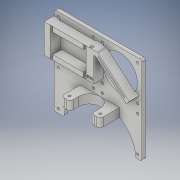
# Autodesk Inventor part: 30_LS_Sample_stage_v2
Saved by Autodesk Inventor 2019 (Build 230136000, 136)
## iProperties
Created: 2020-06-11
Part Number: 30_LS_Sample_stage_v2
Material: Generic
Document SubType Name: Modeling
Designer: UC2
Density: 1 g/cm^3
Appearance: Default
Author: UC2
Autodesk Inventor part; units mm, degrees
ref_plane "YZ Plane" through (0, 0, 0) normal (1, 0, 0) x (0, 1, 0)
ref_plane "XZ Plane" through (0, 0, 0) normal (0, 1, 0) x (-1, 0, 0)
ref_plane "XY Plane" through (0, 0, 0) normal (0, 0, 1) x (1, 0, 0)
sketch "Skizze1" plane through (0, 0, 0) normal (0, 0, 1) x (1, 0, 0)
  line L0 (9.1, 17.5) -> (9.1, 25) construction
  line L1 (9.1, 17.5) -> (15.5, 17.5) construction
  arc A0 (17.5, 15.5) -> (15.5, 17.5) centre (15.5, 15.5) ccw construction
  line L2 (17.5, 15.5) -> (17.5, 9.1) construction
  line L3 (25, 9.1) -> (17.5, 9.1) construction
  line L4 (25, 9.1) -> (25, 25) construction
  line L5 (25, 25) -> (9.1, 25) construction
  circle A1 centre (20, 20) radius 2.2989 construction
  line L6 (-9.1, 25) -> (-9.1, 17.5) construction
  line L7 (-9.1, 25) -> (-25, 25) construction
  line L8 (-25, 25) -> (-25, 9.1) construction
  line L9 (-17.5, 9.1) -> (-25, 9.1) construction
  line L10 (-17.5, 9.1) -> (-17.5, 15.5) construction
  arc A2 (-15.5, 17.5) -> (-17.5, 15.5) centre (-15.5, 15.5) ccw construction
  line L11 (-15.5, 17.5) -> (-9.1, 17.5) construction
  circle A3 centre (-20, 20) radius 2.2989 construction
  circle A4 centre (-20, -20) radius 2.2989 construction
  line L12 (-25, -9.1) -> (-17.5, -9.1) construction
  line L13 (-25, -9.1) -> (-25, -25) construction
  line L14 (-25, -25) -> (-9.1, -25) construction
  line L15 (-9.1, -17.5) -> (-9.1, -25) construction
  line L16 (-9.1, -17.5) -> (-15.5, -17.5) construction
  arc A5 (-17.5, -15.5) -> (-15.5, -17.5) centre (-15.5, -15.5) ccw construction
  line L17 (-17.5, -15.5) -> (-17.5, -9.1) construction
  line L18 (9.1, -25) -> (9.1, -17.5) construction
  line L19 (9.1, -25) -> (25, -25) construction
  line L20 (25, -25) -> (25, -9.1) construction
  line L21 (17.5, -9.1) -> (25, -9.1) construction
  line L22 (17.5, -9.1) -> (17.5, -15.5) construction
  arc A6 (15.5, -17.5) -> (17.5, -15.5) centre (15.5, -15.5) ccw construction
  line L23 (15.5, -17.5) -> (9.1, -17.5) construction
  circle A7 centre (20, -20) radius 2.2989 construction
  circle A8 centre (30, -20) radius 2.2989 construction
  line L24 (25, -9.1) -> (32.5, -9.1) construction
  line L25 (25, -9.1) -> (25, -25) construction
  line L26 (25, -25) -> (40.9, -25) construction
  line L27 (40.9, -17.5) -> (40.9, -25) construction
  line L28 (40.9, -17.5) -> (34.5, -17.5) construction
  arc A9 (32.5, -15.5) -> (34.5, -17.5) centre (34.5, -15.5) ccw construction
  line L29 (32.5, -15.5) -> (32.5, -9.1) construction
  line L30 (40.9, 25) -> (40.9, 17.5) construction
  line L31 (40.9, 25) -> (25, 25) construction
  line L32 (25, 25) -> (25, 9.1) construction
  line L33 (32.5, 9.1) -> (25, 9.1) construction
  line L34 (32.5, 9.1) -> (32.5, 15.5) construction
  arc A10 (34.5, 17.5) -> (32.5, 15.5) centre (34.5, 15.5) ccw construction
  line L35 (34.5, 17.5) -> (40.9, 17.5) construction
  circle A11 centre (30, 20) radius 2.2989 construction
  line L36 (59.1, 17.5) -> (59.1, 25) construction
  line L37 (59.1, 17.5) -> (65.5, 17.5) construction
  arc A12 (67.5, 15.5) -> (65.5, 17.5) centre (65.5, 15.5) ccw construction
  line L38 (67.5, 15.5) -> (67.5, 9.1) construction
  line L39 (75, 9.1) -> (67.5, 9.1) construction
  line L40 (75, 9.1) -> (75, 25) construction
  line L41 (75, 25) -> (59.1, 25) construction
  circle A13 centre (70, 20) radius 2.2989 construction
  line L42 (59.1, -25) -> (59.1, -17.5) construction
  line L43 (59.1, -25) -> (75, -25) construction
  line L44 (75, -25) -> (75, -9.1) construction
  line L45 (67.5, -9.1) -> (75, -9.1) construction
  line L46 (67.5, -9.1) -> (67.5, -15.5) construction
  arc A14 (65.5, -17.5) -> (67.5, -15.5) centre (65.5, -15.5) ccw construction
  line L47 (65.5, -17.5) -> (59.1, -17.5) construction
  circle A15 centre (70, -20) radius 2.2989 construction
  line L48 (213.1196, -154.9196) -> (-182.4616, 240.6616) construction
  line L49 (-24.9, 24.9) -> (74.7, 24.9)
  line L50 (74.7, 24.9) -> (74.7, -74.7)
  line L51 (74.7, -74.7) -> (-24.9, -74.7)
  line L52 (-24.9, -74.7) -> (-24.9, 24.9)
  circle A16 centre (50, 0) radius 19.7246
  point P0 (0, 0)
  dimension "d0" = 99.6
  dimension "d1" = 99.6
  dimension "d2" = 0.1
  dimension "d3" = 0.1
  constraints: 10 end point, 2 parallel, 1 coincident, 1 horizontal, 1 perpendicular, 6 other
  measures "d0" distance of L51.end L49.start
  measures "d1" distance of L50.end L51.end
  measures "d2" distance between parallel lines of L8 L52
  measures "d3" distance between parallel lines of L7 L49
extrude "Extrusion1" add sketch "Skizze1" along normal blind 4
sketch "Skizze2" plane through (0, 0, 0) normal (0, 0, -1) x (-1, 0, 0)
  circle A0 centre (20, -20) radius 2.1796 construction
  circle A1 centre (20, 20) radius 2.1796 construction
  circle A2 centre (-20, 20) radius 2.1796 construction
  circle A3 centre (-20, -20) radius 2.1796 construction
  circle A4 centre (-30, -20) radius 2.1796 construction
  circle A5 centre (-70, -20) radius 2.1796 construction
  circle A6 centre (-70, 20) radius 2.1796 construction
  circle A7 centre (-30, 20) radius 2.1796 construction
  circle A8 centre (-70, -70) radius 2.65 construction
  circle A9 centre (-30, -70) radius 2.65 construction
  circle A10 centre (-20, -70) radius 2.65 construction
  circle A11 centre (20, -70) radius 2.65 construction
  circle A12 centre (20, -30) radius 2.65 construction
  circle A13 centre (-20, -30) radius 2.65 construction
  circle A14 centre (-30, -30) radius 2.65 construction
  circle A15 centre (-70, -30) radius 2.65 construction
  point P0 (0, 0)
hole "Bohrung1" at (-20, -20, 0) at (-20, 20, 0) at (20, -20, 0) at (30, -20, 0) at (70, -20, 0) at (70, 20, 0) at (30, 20, 0) at (20, 20, 0) at (70, -30, 0) at (30, -30, 0) at (20, -30, 0) at (-20, -30, 0) at (-20, -70, 0) at (20, -70, 0) at (30, -70, 0) at (70, -70, 0) direction (0, 0, 1) diameter 2.8 end through all
ref_plane "Arbeitsebene1" through (0, 0, 5.25) normal (0, 0, 1) x (1, 0, 0)
sketch "Skizze4" plane through (0, 0, 5.25) normal (0, 0, 1) x (1, 0, 0)
  line L0 (-24.9, 24.9) -> (-24.9, -74.7) construction
  line L1 (-24.9, -74.7) -> (74.7, -74.7) construction
  line L2 (74.7, -74.7) -> (74.7, 24.9) construction
  line L3 (74.7, 24.9) -> (-24.9, 24.9) construction
  circle A0 centre (30, 20) radius 1.4 construction
  circle A1 centre (70, -20) radius 1.4 construction
  circle A2 centre (20, -20) radius 1.4 construction
  circle A3 centre (-20, -20) radius 1.4 construction
  circle A4 centre (-20, 20) radius 1.4 construction
  circle A5 centre (30, -20) radius 1.4 construction
  circle A6 centre (70, 20) radius 1.4 construction
  circle A7 centre (20, 20) radius 1.4 construction
  circle A8 centre (51.5846, 1.8884) radius 19.7246 construction
  circle A9 centre (70, -20) radius 1.4 construction
  line L4 (-24.9, 18.6) -> (-17.9, 18.6)
  line L5 (-17.9, 18.6) -> (-17.9, -14.4)
  line L6 (-17.9, -14.4) -> (-24.9, -14.4)
  line L7 (-24.9, -14.4) -> (-24.9, 18.6)
  line L8 (31.6685, 18.6) -> (22.6685, 18.6)
  line L9 (22.6685, 18.6) -> (22.6685, -14.4)
  line L10 (22.6685, -14.4) -> (31.6685, -14.4)
  line L11 (31.6685, -14.4) -> (31.6685, 18.6)
  line L12 (-17.9, 18.6) -> (22.6685, 18.6)
  line L13 (22.6685, 18.6) -> (22.6685, 18.1)
  line L14 (22.6685, 18.1) -> (-17.9, 18.1)
  line L15 (-17.9, 18.1) -> (-17.9, 18.6)
  line L16 (-17.9, -14.4) -> (22.6685, -14.4)
  line L17 (22.6685, -14.4) -> (22.6685, -13.9)
  line L18 (22.6685, -13.9) -> (-17.9, -13.9)
  line L19 (-17.9, -13.9) -> (-17.9, -14.4)
  line L20 (-14.9, -13.9) -> (19.6685, -13.9)
  line L21 (19.6685, -13.9) -> (19.6685, -8.9)
  line L22 (19.6685, -8.9) -> (-14.9, -8.9)
  line L23 (-14.9, -8.9) -> (-14.9, -13.9)
  line L24 (-14.9, 18.1) -> (19.6685, 18.1)
  line L25 (19.6685, 18.1) -> (19.6685, 13.1)
  line L26 (19.6685, 13.1) -> (-14.9, 13.1)
  line L27 (-14.9, 13.1) -> (-14.9, 18.1)
  line L28 (22.6685, 18.6) -> (31.6685, 18.6)
  line L29 (31.6685, 18.6) -> (31.6685, -14.4)
  line L30 (31.6685, -14.4) -> (22.6685, -14.4)
  line L31 (22.6685, -14.4) -> (22.6685, 18.6)
  line L32 (30, 20) -> (73.3204, -16.3501) construction
  line L33 (31.6685, 18.6) -> (34.9854, 18.6)
  line L34 (36.271, 18.1321) -> (71.6704, -11.5715)
  line L35 (71.6704, -11.5715) -> (68.3279, -15.555)
  line L36 (68.3279, -15.555) -> (34.14, 13.1321)
  line L37 (32.8544, 13.6) -> (31.6685, 13.6)
  line L38 (66.3088, -11.25) -> (36.089, 14.1075)
  line L39 (36.089, 14.1075) -> (36.8603, 15.0268)
  line L40 (36.8603, 15.0268) -> (67.0802, -10.3307)
  line L41 (67.0802, -10.3307) -> (66.3088, -11.25)
  line L42 (66.3088, -11.25) -> (36.8603, 15.0268) construction
  line L43 (36.089, 14.1075) -> (67.0802, -10.3307) construction
  arc A10 (34.14, 13.1321) -> (32.8544, 13.6) centre (32.8544, 11.6) ccw
  arc A11 (36.271, 18.1321) -> (34.9854, 18.6) centre (34.9854, 16.6) ccw
  line L44 (31.6685, 13.6) -> (31.6685, 18.6)
  line L45 (30, 20) -> (70, 20) construction
  point P0 (0, 0)
  point P1 (51.5846, 1.8884)
  dimension "d15" = 5
  dimension "d16" = 5
  dimension "d17" = 3
  dimension "d18" = 3
  dimension "d19" = 0.5
  dimension "d20" = 0.5
  dimension "d21" = 7
  dimension "d22" = 9
  dimension "d70" = 33
  dimension "d71" = 5
  dimension "d73" = 1.2
  dimension "d74" = 2
  dimension "d75" = 5.2
  dimension "d95" = 40
  constraints: 84 end point, 20 parallel, 12 point on line, 9 horizontal, 9 perpendicular, 5 tangent, 4 point on circle, 3 centre point, 3 midpoint, 1 coincident, 1 collinear, 1 equal radius, 1 other
  measures "d15" distance of L26.end L24.start
  measures "d16" distance of L22.end L20.start
  measures "d17" distance between parallel lines of L5 L23
  measures "d18" distance between parallel lines of L9 L21
  measures "d19" distance between parallel lines of L16 L18
  measures "d20" distance between parallel lines of L14 L12
  measures "d21" distance of L4.start L4.end
  measures "d22" distance of L8.start L8.end
  measures "d70" distance of L4.end L5.end
  measures "d71" distance between parallel lines of L33 L37
  measures "d73" distance of L38.end L39.end
  measures "d74" radius of A10
  measures "d75" distance of L34.end L35.end
  measures "d95" angle of L32 L45
extrude "Extrusion2" add sketch "Skizze4" along normal blind 20 contours L4 L5 L6 L7 | L12 L9 L14 L5 | L8 L11 L10 L9 | L5 L18 L9 L16 | L14 L25 L26 L27 | L33 A11 L34 L35 L36 A10 L37 L11 | L23 L22 L21 L18
sketch "Skizze5" plane through (0, 0, 4) normal (0, 0, 1) x (1, 0, 0)
  line L0 (-24.9, -14.4) -> (31.6685, -14.4) construction
  line L1 (34.9854, 18.6) -> (-24.9, 18.6) construction
  line L2 (-24.9, 18.6) -> (-24.9, -14.4) construction
  line L3 (-17.9, -13.9) -> (-17.9, 18.1) construction
  line L4 (-17.9, 18.1) -> (-14.9, 18.1) construction
  line L5 (-14.9, 18.1) -> (-14.9, 13.1) construction
  line L6 (-14.9, 13.1) -> (19.6685, 13.1) construction
  line L7 (19.6685, 13.1) -> (19.6685, 18.1) construction
  line L8 (19.6685, 18.1) -> (22.6685, 18.1) construction
  line L9 (22.6685, -13.9) -> (19.6685, -13.9) construction
  line L10 (19.6685, -13.9) -> (19.6685, -8.9) construction
  line L11 (19.6685, -8.9) -> (-14.9, -8.9) construction
  line L12 (-14.9, -8.9) -> (-14.9, -13.9) construction
  line L13 (-14.9, -13.9) -> (-17.9, -13.9) construction
  line L14 (-24.9, 18.6) -> (-17.9, 18.6)
  line L15 (-17.9, 18.6) -> (-17.9, -14.4)
  line L16 (-17.9, -14.4) -> (-24.9, -14.4)
  line L17 (-24.9, -14.4) -> (-24.9, 18.6)
  line L18 (31.6685, -14.4) -> (31.6685, 13.6) projected
  line L19 (22.6685, 18.1) -> (22.6685, -13.9) projected
  line L20 (31.6685, 13.6) -> (32.8544, 13.6) projected
  arc A0 (34.14, 13.1321) -> (32.8544, 13.6) centre (32.8544, 11.6) ccw projected
  line L21 (34.14, 13.1321) -> (68.3279, -15.555) projected
  line L22 (68.3279, -15.555) -> (71.6704, -11.5715) projected
  line L23 (71.6704, -11.5715) -> (36.271, 18.1321) projected
  arc A1 (36.271, 18.1321) -> (34.9854, 18.6) centre (34.9854, 16.6) ccw projected
  point P0 (0, 0)
  constraints: 8 end point, 2 parallel, 1 horizontal, 1 perpendicular, 1 point on line
extrude "Extrusion3" add sketch "Skizze5" along normal up to next
sketch "Skizze9" plane through (0, 0, 4) normal (0, 0, 1) x (1, 0, 0)
  line L0 (74.7, -74.7) -> (74.7, 24.9) construction
  line L1 (74.7, 24.9) -> (-24.9, 24.9) construction
  line L2 (-24.9, -14.4) -> (-24.9, -74.7) construction
  line L3 (-24.9, 18.6) -> (-20, 18.6) construction
  line L4 (-17.9, 18.6) -> (-17.9, -14.4) construction
  line L5 (-17.9, -14.4) -> (-24.9, -14.4) construction
  line L6 (-24.9, 24.9) -> (-24.9, 18.6) construction
  circle A0 centre (30, 20) radius 1.4 construction
  circle A1 centre (70, -20) radius 1.4 construction
  circle A2 centre (20, -20) radius 1.4 construction
  circle A3 centre (-20, -20) radius 1.4 construction
  circle A4 centre (-20, 20) radius 1.4 construction
  circle A5 centre (30, -20) radius 1.4 construction
  circle A6 centre (70, 20) radius 1.4 construction
  circle A7 centre (20, 20) radius 1.4 construction
  circle A8 centre (50, 0) radius 19.7246 construction
  line L7 (34.9854, 18.6) -> (-24.9, 18.6) construction
  line L8 (-24.9, 18.6) -> (-24.9, -14.4) construction
  line L9 (-24.9, -14.4) -> (31.6685, -14.4) construction
  line L10 (-17.9, 18.1) -> (-14.9, 18.1) construction
  line L11 (-14.9, 18.1) -> (-14.9, 13.1) construction
  line L12 (-14.9, 13.1) -> (19.6685, 13.1) construction
  line L13 (19.6685, 13.1) -> (19.6685, 18.1) construction
  line L14 (19.6685, 18.1) -> (22.6685, 18.1) construction
  line L15 (22.6685, -13.9) -> (19.6685, -13.9) construction
  line L16 (19.6685, -13.9) -> (19.6685, -8.9) construction
  line L17 (19.6685, -8.9) -> (-14.9, -8.9) construction
  line L18 (-14.9, -8.9) -> (-14.9, -13.9) construction
  line L19 (-14.9, -13.9) -> (-17.9, -13.9) construction
  line L20 (-17.9, -13.9) -> (-17.9, 18.1) construction
  line L21 (5.1685, -34.4) -> (49.1685, -34.4)
  line L22 (49.1685, -34.4) -> (49.1685, -44.4)
  line L23 (49.1685, -44.4) -> (5.1685, -44.4)
  line L24 (5.1685, -44.4) -> (5.1685, -34.4)
  line L25 (31.6685, -14.4) -> (31.6685, 13.6) projected
  line L26 (22.6685, 18.1) -> (22.6685, -13.9) projected
  line L27 (-20, 18.6) -> (-17.9, 18.6) projected
  line L28 (31.6685, 13.6) -> (32.8544, 13.6) projected
  arc A9 (34.14, 13.1321) -> (32.8544, 13.6) centre (32.8544, 11.6) ccw projected
  line L29 (34.14, 13.1321) -> (68.3279, -15.555) projected
  line L30 (68.3279, -15.555) -> (71.6704, -11.5715) projected
  line L31 (71.6704, -11.5715) -> (36.271, 18.1321) projected
  arc A10 (36.271, 18.1321) -> (34.9854, 18.6) centre (34.9854, 16.6) ccw projected
  line L32 (27.1685, 18.6) -> (27.1685, -74.7) construction
  line L33 (74.7, -74.7) -> (-24.9, -74.7) construction
  line L34 (-24.9, -74.7) -> (74.7, -74.7) projected
  point P0 (0, 0)
  dimension "d44" = 10
  dimension "d45" = 20
  dimension "d53" = 44
  dimension "d80" = 4.5
  constraints: 10 end point, 2 parallel, 2 point on line, 1 horizontal, 1 perpendicular, 1 vertical, 1 vertical alignment, 1 other
  measures "d44" distance of L23.end L21.start
  measures "d45" distance between parallel lines of L9 L21
  measures "d53" distance of L22.end L23.end
  measures "d80" distance between parallel lines of L26 L32
extrude "Extrusion6" add sketch "Skizze9" along normal blind 22
sketch "Skizze10" plane through (5.1685, -44.4, 4) normal (0, -1, 0) x (1, 0, 0)
  circle A0 centre (4.5, 17) radius 2.1 construction
  circle A1 centre (39.5, 17) radius 2.1 construction
  circle A2 centre (22, 6.652) radius 4.55 construction
  circle A3 centre (4.5, 17) radius 1.4
  circle A4 centre (39.5, 17) radius 1.4
  line L0 (29.8169, 1.25) -> (-23.0685, 1.25) projected
  line L1 (44, 0) -> (0, 0) construction
  line L2 (44, 0) -> (44, 22) construction
  line L3 (0, 22) -> (44, 22) construction
  line L4 (0, 0) -> (0, 22) construction
  line L5 (0, 22) -> (44, 22) construction
  line L6 (22, 22) -> (22, -2.1382) construction
  line L7 (22, 12) -> (22, 21.4772) construction
  line L8 (34, 12) -> (34, 21.4772)
  line L9 (10, 21.4772) -> (10, 12)
  arc A5 (10, 12) -> (34, 12) centre (22, 12) ccw
  arc A6 (34, 21.4772) -> (10, 21.4772) centre (22, 21.4772) ccw
  point P0 (-5.1685, -4)
  point P1 (56.4063, 1.25)
  point P2 (3.1, 1.25)
  point P3 (22, 16.7386)
  point P4 (50.2492, 1.25)
  point P5 (4.1, 1.25)
  dimension "d48" = 2.8
  dimension "d49" = 2.8
  dimension "d54" = 35
  dimension "d65" = 24
  dimension "d78" = 5
  constraints: 10 end point, 7 centre point, 5 tangent, 4 point on circle, 3 point on line, 2 coincident, 2 midpoint, 1 parallel, 1 perpendicular, 1 symmetric about line
  measures "d48" diameter of A3
  measures "d49" diameter of A4
  measures "d54" distance of A0.centre A1.centre
  measures "d65" distance between parallel lines of L9 L8
  measures "d78" distance from line of L3 A0.centre
extrude "Extrusion7" cut sketch "Skizze10" against normal up to surface (10 mm away)
fillet "Rundung3" radius 3.5 4 edges at (49.1685, -39.4, 26) (5.1685, -39.4, 26) (15.1798, -39.4, 26) (39.1571, -39.4, 26)
sketch "Skizze15" plane through (-17.9, -14.4, 5.25) normal (0, -1, 0) x (1, 0, 0)
  line L0 (0, -1.25) -> (0, 0) construction
  line L1 (0, 0) -> (49.5685, 0) construction
  line L2 (49.5685, 0) -> (49.5685, 20) construction
  line L3 (-7, 20) -> (49.5685, 20) construction
  line L4 (-7, -1.25) -> (-7, 20) projected
  line L5 (0, -1.25) -> (-7, -1.25) projected
  line L6 (44.7786, 9.164) -> (46.148, 8.708) construction
  line L7 (46.148, 8.708) -> (46.4379, 7.2941) construction
  line L8 (46.4379, 7.2941) -> (45.3583, 6.336) construction
  line L9 (45.3583, 6.336) -> (43.9889, 6.792) construction
  line L10 (43.9889, 6.792) -> (43.699, 8.2059) construction
  line L11 (43.699, 8.2059) -> (44.7786, 9.164) construction
  circle A0 centre (45.0685, 7.75) radius 2.45 construction
  point P0 (17.9, -5.25)
hole "Bohrung3" at (27.1685, -14.4, 13) direction (0, 1, 0) diameter 3.5 end through all
sketch "Skizze16" plane through (0, 0, 25.25) normal (0, 0, 1) x (1, 0, 0)
  line L0 (25.4185, 18.6) -> (25.4185, -14.4) construction
  line L1 (28.9185, 18.6) -> (28.9185, -14.4) construction
  line L2 (-17.9, 18.1) -> (-14.9, 18.1) construction
  line L3 (-14.9, 18.1) -> (-14.9, 13.1) construction
  line L4 (-14.9, 13.1) -> (19.6685, 13.1) construction
  line L5 (19.6685, 13.1) -> (19.6685, 18.1) construction
  line L6 (19.6685, 18.1) -> (22.6685, 18.1) construction
  line L7 (22.6685, 18.1) -> (22.6685, -13.9) construction
  line L8 (22.6685, -13.9) -> (19.6685, -13.9) construction
  line L9 (19.6685, -13.9) -> (19.6685, -8.9) construction
  line L10 (19.6685, -8.9) -> (-14.9, -8.9) construction
  line L11 (-14.9, -8.9) -> (-14.9, -13.9) construction
  line L12 (-14.9, -13.9) -> (-17.9, -13.9) construction
  line L13 (-17.9, -13.9) -> (-17.9, 18.1) construction
  line L14 (36.089, 14.1075) -> (36.8603, 15.0268) construction
  line L15 (36.8603, 15.0268) -> (67.0802, -10.3307) construction
  line L16 (67.0802, -10.3307) -> (66.3088, -11.25) construction
  line L17 (66.3088, -11.25) -> (36.089, 14.1075) construction
  line L18 (34.9854, 18.6) -> (-24.9, 18.6) construction
  line L19 (-24.9, -14.4) -> (31.6685, -14.4) construction
  line L20 (31.6685, -14.4) -> (31.6685, 13.6) construction
  line L21 (31.6685, 13.6) -> (32.8544, 13.6) construction
  arc A0 (34.14, 13.1321) -> (32.8544, 13.6) centre (32.8544, 11.6) ccw construction
  line L22 (34.14, 13.1321) -> (68.3279, -15.555) construction
  line L23 (68.3279, -15.555) -> (71.6704, -11.5715) construction
  line L24 (71.6704, -11.5715) -> (36.271, 18.1321) construction
  arc A1 (36.271, 18.1321) -> (34.9854, 18.6) centre (34.9854, 16.6) ccw construction
  line L25 (28.9185, -14.4) -> (25.4185, -14.4) projected
  line L26 (27.1685, -14.4) -> (27.1685, 18.6) construction
  line L27 (34.9854, 18.6) -> (-24.9, 18.6) projected
  line L28 (23.9185, -11.8716) -> (30.4185, -11.8716)
  line L29 (30.4185, -11.8716) -> (30.4185, -9.3716)
  line L30 (30.4185, -9.3716) -> (23.9185, -9.3716)
  line L31 (23.9185, -9.3716) -> (23.9185, -11.8716)
  line L32 (-24.9, 18.6) -> (-24.9, -14.4) projected
  point P0 (0, 0)
  dimension "d88" = 2.5
  dimension "d89" = 6.5
  constraints: 10 end point, 2 parallel, 2 perpendicular, 1 horizontal, 1 midpoint, 1 point on line, 1 other
  measures "d88" distance of L28.end L29.end
  measures "d89" distance of L28.start L28.end
extrude "Extrusion12" cut sketch "Skizze16" against normal up to surface (21.25 mm away)
sketch "Skizze17" plane through (0, 0, 25.25) normal (0, 0, 1) x (1, 0, 0)
  line L0 (30.4185, -11.8716) -> (23.9185, -11.8716) construction
  line L1 (23.9185, -11.8716) -> (23.9185, -9.3716) construction
  line L2 (23.9185, -9.3716) -> (30.4185, -9.3716) construction
  line L3 (30.4185, -9.3716) -> (30.4185, -11.8716) construction
  line L4 (-17.9, 18.1) -> (-14.9, 18.1) construction
  line L5 (-14.9, 18.1) -> (-14.9, 13.1) construction
  line L6 (-14.9, 13.1) -> (19.6685, 13.1) construction
  line L7 (19.6685, 13.1) -> (19.6685, 18.1) construction
  line L8 (19.6685, 18.1) -> (22.6685, 18.1) construction
  line L9 (22.6685, 18.1) -> (22.6685, -13.9) construction
  line L10 (22.6685, -13.9) -> (19.6685, -13.9) construction
  line L11 (19.6685, -13.9) -> (19.6685, -8.9) construction
  line L12 (19.6685, -8.9) -> (-14.9, -8.9) construction
  line L13 (-14.9, -8.9) -> (-14.9, -13.9) construction
  line L14 (-14.9, -13.9) -> (-17.9, -13.9) construction
  line L15 (-17.9, -13.9) -> (-17.9, 18.1) construction
  line L16 (36.089, 14.1075) -> (36.8603, 15.0268) construction
  line L17 (36.8603, 15.0268) -> (67.0802, -10.3307) construction
  line L18 (67.0802, -10.3307) -> (66.3088, -11.25) construction
  line L19 (66.3088, -11.25) -> (36.089, 14.1075) construction
  line L20 (34.9854, 18.6) -> (-24.9, 18.6) construction
  line L21 (-24.9, -14.4) -> (31.6685, -14.4) construction
  line L22 (31.6685, -14.4) -> (31.6685, 13.6) construction
  line L23 (31.6685, 13.6) -> (32.8544, 13.6) construction
  arc A0 (34.14, 13.1321) -> (32.8544, 13.6) centre (32.8544, 11.6) ccw construction
  line L24 (34.14, 13.1321) -> (68.3279, -15.555) construction
  line L25 (68.3279, -15.555) -> (71.6704, -11.5715) construction
  line L26 (71.6704, -11.5715) -> (36.271, 18.1321) construction
  arc A1 (36.271, 18.1321) -> (34.9854, 18.6) centre (34.9854, 16.6) ccw construction
  line L27 (34.9854, 18.6) -> (-17.9, 18.6) projected
  line L28 (31.6685, 18.6) -> (74.3161, 18.6)
  line L29 (74.3161, 18.6) -> (74.3161, -17.9689)
  line L30 (74.3161, -17.9689) -> (31.6685, -17.9689)
  line L31 (31.6685, -17.9689) -> (31.6685, 18.6)
  line L32 (-24.9, 18.6) -> (-24.9, -14.4) projected
  line L33 (31.6685, 18.6) -> (-45.9766, 18.6)
  line L34 (-45.9766, 18.6) -> (-45.9766, -17.9689)
  line L35 (-45.9766, -17.9689) -> (31.6685, -17.9689)
  line L36 (31.6685, -17.9689) -> (31.6685, 18.6)
  point P0 (0, 0)
  constraints: 16 end point, 4 parallel, 2 horizontal, 2 perpendicular, 2 point on line
extrude "Extrusion13" cut sketch "Skizze17" against normal blind 10
sketch "Skizze18" plane through (0, 0, 4) normal (0, 0, 1) x (1, 0, 0)
  line L0 (49.1685, -34.4) -> (49.1685, -44.4) construction
  line L1 (49.1685, -44.4) -> (27.1685, -44.4) construction
  line L2 (27.1685, -44.4) -> (5.1685, -44.4) construction
  line L3 (5.1685, -44.4) -> (5.1685, -34.4) construction
  line L4 (5.1685, -34.4) -> (27.1685, -34.4) construction
  line L5 (27.1685, -34.4) -> (49.1685, -34.4) construction
  circle A0 centre (50, 0) radius 19.7246 construction
  circle A1 centre (70, -70) radius 1.4 construction
  circle A2 centre (20, -70) radius 1.4 construction
  circle A3 centre (-20, -30) radius 1.4 construction
  circle A4 centre (30, -30) radius 1.4 construction
  circle A5 centre (20, 20) radius 1.4 construction
  circle A6 centre (70, 20) radius 1.4 construction
  circle A7 centre (30, -20) radius 1.4 construction
  line L6 (-24.9, 24.9) -> (-24.9, 18.6) construction
  circle A8 centre (-20, 20) radius 1.4 construction
  line L7 (-24.9, -14.4) -> (-24.9, -74.7) construction
  line L8 (-24.9, -74.7) -> (74.7, -74.7) construction
  line L9 (74.7, -74.7) -> (74.7, 24.9) construction
  line L10 (74.7, 24.9) -> (-24.9, 24.9) construction
  circle A9 centre (-20, -20) radius 1.4 construction
  circle A10 centre (20, -20) radius 1.4 construction
  circle A11 centre (70, -20) radius 1.4 construction
  circle A12 centre (30, 20) radius 1.4 construction
  circle A13 centre (70, -30) radius 1.4 construction
  circle A14 centre (20, -30) radius 1.4 construction
  circle A15 centre (-20, -70) radius 1.4 construction
  circle A16 centre (30, -70) radius 1.4 construction
  line L11 (13.1685, -63.9) -> (41.1685, -63.9) construction
  circle A17 centre (27.1685, -74.7) radius 40.5 construction
  line L12 (5.1685, -44.4) -> (49.1685, -44.4)
  line L13 (-13.3315, -74.7) -> (67.6685, -74.7)
  arc A18 (5.1685, -44.4) -> (-13.3315, -74.7) centre (20.7317, -74.7) ccw
  arc A19 (67.6685, -74.7) -> (49.1685, -44.4) centre (33.6052, -74.7) ccw
  line L14 (27.1685, -44.4) -> (27.1685, -74.7) construction
  line L15 (72.7, -74.7) -> (-22.9, -74.7) construction
  line L16 (-24.9, 18.6) -> (-20, 18.6) projected
  line L17 (-20, 18.6) -> (-17.9, 18.6) projected
  line L18 (-17.9, 18.6) -> (-17.9, -14.4) projected
  line L19 (-17.9, -14.4) -> (-24.9, -14.4) projected
  point P0 (0, 0)
  dimension "d97" = 81
  constraints: 6 end point, 6 point on circle, 3 centre point, 3 point on line, 2 collinear, 2 horizontal, 2 tangent, 1 vertical, 1 vertical alignment
  measures "d97" diameter of A17
extrude "Extrusion14" cut sketch "Skizze18" against normal through all
fillet "Rundung6" radius 2 6 edges at (74.7, -74.7, 2) (67.6685, -74.7, 2) (-13.3315, -74.7, 2) (-24.9, -74.7, 2) (74.7, 24.9, 2) (-24.9, 24.9, 2)
sketch "Skizze21" plane through (0, 0, 4) normal (0, 0, 1) x (1, 0, 0)
  arc A0 (-22.9, 24.9) -> (-24.9, 22.9) centre (-22.9, 22.9) ccw construction
  line L0 (-24.9, 22.9) -> (-24.9, 18.6) construction
  line L1 (-24.9, 18.6) -> (-20, 18.6) construction
  circle A1 centre (-20, 20) radius 1.4 construction
  line L2 (-20, 18.6) -> (-17.9, 18.6) construction
  line L3 (-17.9, 18.6) -> (-17.9, -14.4) construction
  line L4 (-17.9, -14.4) -> (-24.9, -14.4) construction
  line L5 (-24.9, -14.4) -> (-24.9, -72.7) construction
  arc A2 (-24.9, -72.7) -> (-22.9, -74.7) centre (-22.9, -72.7) ccw construction
  line L6 (-22.9, -74.7) -> (-15.276, -74.7) construction
  arc A3 (-15.276, -74.7) -> (-13.2791, -72.8109) centre (-15.276, -72.7) ccw construction
  arc A4 (5.1685, -44.4) -> (-13.2791, -72.8109) centre (20.7317, -74.7) ccw construction
  line L7 (5.1685, -44.4) -> (5.1685, -34.4) construction
  line L8 (5.1685, -34.4) -> (27.1685, -34.4) construction
  line L9 (27.1685, -34.4) -> (49.1685, -34.4) construction
  line L10 (49.1685, -34.4) -> (49.1685, -44.4) construction
  arc A5 (67.616, -72.8109) -> (49.1685, -44.4) centre (33.6052, -74.7) ccw construction
  arc A6 (67.616, -72.8109) -> (69.613, -74.7) centre (69.613, -72.7) ccw construction
  line L11 (69.613, -74.7) -> (72.7, -74.7) construction
  arc A7 (72.7, -74.7) -> (74.7, -72.7) centre (72.7, -72.7) ccw construction
  line L12 (74.7, -72.7) -> (74.7, 22.9) construction
  arc A8 (74.7, 22.9) -> (72.7, 24.9) centre (72.7, 22.9) ccw construction
  line L13 (72.7, 24.9) -> (-22.9, 24.9) construction
  circle A9 centre (-20, -70) radius 1.4 construction
  circle A10 centre (20, -30) radius 1.4 construction
  circle A11 centre (70, -30) radius 1.4 construction
  circle A12 centre (30, 20) radius 1.4 construction
  circle A13 centre (70, -20) radius 1.4 construction
  circle A14 centre (20, -20) radius 1.4 construction
  circle A15 centre (-20, -20) radius 1.4 construction
  circle A16 centre (30, -20) radius 1.4 construction
  circle A17 centre (70, 20) radius 1.4 construction
  circle A18 centre (20, 20) radius 1.4 construction
  circle A19 centre (30, -30) radius 1.4 construction
  circle A20 centre (-20, -30) radius 1.4 construction
  circle A21 centre (70, -70) radius 1.4 construction
  circle A22 centre (50, 0) radius 19.7246 construction
  arc A23 (36.271, 18.1321) -> (34.9854, 18.6) centre (34.9854, 16.6) ccw construction
  line L14 (-24.9, 18.6) -> (34.9854, 18.6) construction
  line L15 (-24.9, -14.4) -> (-24.9, 18.6) construction
  line L16 (31.6685, -14.4) -> (-24.9, -14.4) construction
  line L17 (31.6685, 13.6) -> (31.6685, -14.4) construction
  line L18 (32.8544, 13.6) -> (31.6685, 13.6) construction
  arc A24 (34.14, 13.1321) -> (32.8544, 13.6) centre (32.8544, 11.6) ccw construction
  line L19 (68.3279, -15.555) -> (34.14, 13.1321) construction
  line L20 (71.6704, -11.5715) -> (68.3279, -15.555) construction
  line L21 (36.271, 18.1321) -> (71.6704, -11.5715) construction
  line L22 (36.8603, 15.0268) -> (36.089, 14.1075) construction
  line L23 (67.0802, -10.3307) -> (36.8603, 15.0268) construction
  line L24 (66.3088, -11.25) -> (67.0802, -10.3307) construction
  line L25 (36.089, 14.1075) -> (66.3088, -11.25) construction
  line L26 (19.6685, 18.1) -> (19.6685, 13.1) construction
  line L27 (22.6685, 18.1) -> (19.6685, 18.1) construction
  line L28 (22.6685, -13.9) -> (22.6685, 18.1) construction
  line L29 (19.6685, -13.9) -> (22.6685, -13.9) construction
  line L30 (19.6685, -8.9) -> (19.6685, -13.9) construction
  line L31 (-14.9, -8.9) -> (19.6685, -8.9) construction
  line L32 (-14.9, -13.9) -> (-14.9, -8.9) construction
  line L33 (-17.9, -13.9) -> (-14.9, -13.9) construction
  line L34 (-17.9, 18.1) -> (-17.9, -13.9) construction
  line L35 (-14.9, 18.1) -> (-17.9, 18.1) construction
  line L36 (-14.9, 13.1) -> (-14.9, 18.1) construction
  line L37 (19.6685, 13.1) -> (-14.9, 13.1) construction
  line L38 (23.9185, -9.3716) -> (23.9185, -11.8716) construction
  line L39 (30.4185, -9.3716) -> (23.9185, -9.3716) construction
  line L40 (30.4185, -11.8716) -> (30.4185, -9.3716) construction
  line L41 (23.9185, -11.8716) -> (30.4185, -11.8716) construction
  line L42 (31.6685, -14.4) -> (22.6685, -14.4)
  line L43 (22.6685, -14.4) -> (22.6685, 18.6)
  line L44 (22.6685, 18.6) -> (31.6685, 18.6)
  line L45 (31.6685, 18.6) -> (31.6685, -14.4)
  line L46 (31.0685, -13.8) -> (23.2685, -13.8)
  line L47 (23.2685, -13.8) -> (23.2685, 18)
  line L48 (23.2685, 18) -> (31.0685, 18)
  line L49 (31.0685, 18) -> (31.0685, -13.8)
  line L50 (71.6704, -11.5715) -> (68.3279, -15.555)
  line L51 (68.3279, -15.555) -> (65.0232, -12.782)
  line L52 (65.0232, -12.782) -> (68.3657, -8.7986)
  line L53 (68.3657, -8.7986) -> (71.6704, -11.5715)
  line L54 (68.4397, -9.6439) -> (65.8685, -12.7081)
  line L55 (65.8685, -12.7081) -> (68.2539, -14.7097)
  line L56 (68.2539, -14.7097) -> (70.8251, -11.6455)
  line L57 (70.8251, -11.6455) -> (68.4397, -9.6439)
  point P0 (0, 0)
  dimension "d101" = 0.6
  dimension "d102" = 0.6
  constraints: 32 end point, 9 equal length, 4 perpendicular, 2 point on line, 1 horizontal, 1 vertical alignment, 6 other
  measures "d101" distance between parallel lines of L45 L49
  measures "d102" distance between parallel lines of L52 L54
extrude "Extrusion15" add sketch "Skizze21" along normal up to surface (1.25 mm away)
equation "\"d16\" = d15"
equation "\"d18\" = d17"
equation "\"d20\" = d19"
equation "\"d71\" = d15"
equation "\"d80\" = 0.5 * d22"
equation "\"d49\" = d48"
